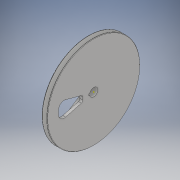
# Autodesk Inventor part: Součást6
Saved by Autodesk Inventor 2019 (Build 230136000, 136)
## iProperties
Created: 2019-10-22
Part Number: Součást6
Material: Všeobecné
Document SubType Name: Modeling
Designer: micaf
Density: 1 g/cm^3
Appearance: Výchozí
Author: micaf
Autodesk Inventor part; units mm, degrees
ref_plane "YZ Plane" through (0, 0, 0) normal (1, 0, 0) x (0, 1, 0)
ref_plane "XY Plane" through (0, 0, 0) normal (0, 0, 1) x (1, 0, 0)
sketch "Náčrt1" plane through (0, 0, 0) normal (0, 0, 1) x (1, 0, 0)
  line L0 (0, -53.3418) -> (0, 320.0509) projected
  line L1 (-48, 0) -> (8, 0) projected
  line L2 (0, 250) -> (0, 0)
  line L3 (0, 0) -> (-40, 0)
  line L4 (-40, 0) -> (-40, 30)
  line L5 (-40, 30) -> (-15, 30)
  line L6 (-15, 30) -> (-15, 210)
  line L7 (-15, 210) -> (-30, 210)
  line L8 (-30, 210) -> (-30, 250)
  line L9 (-26.5993, 250) -> (-17.5, 225)
  line L10 (-17.5, 225) -> (-12.5, 225)
  line L11 (-15, 225) -> (-15, 266.7091) construction
  line L12 (-12.5, 225) -> (-3.4007, 250)
  line L13 (-30, 250) -> (-26.5993, 250)
  line L14 (-3.4007, 250) -> (0, 250)
  dimension "d0" = 30
  dimension "d1" = 40
  dimension "d2" = 15
  dimension "d3" = 250
  dimension "d14" = 30
  dimension "d15" = 15
  dimension "d16" = 20
  dimension "d17" = 20
  dimension "d18" = 25
  dimension "d19" = 40
  dimension "d23" = 5
  dimension "d24" = 15
  constraints: 26 end point, 3 perpendicular, 3 vertical, 2 collinear, 2 horizontal, 2 point on line, 1 midpoint
  measures "d0" distance of L3.end L4.end
  measures "d1" distance of L2.end L3.end
  measures "d2" distance between parallel lines of L2 L6
  measures "d3" distance of L2.start L2.end
  measures "d14" distance of L2.start L8.end
  measures "d15" distance from line of L11 L2.start
  measures "d16" angle of L11 L12
  measures "d17" angle of L9 L11
  measures "d18" vertical distance of L8.end L9.end
  measures "d19" distance of L7.end L8.end
  measures "d23" distance of L9.end L10.end
  measures "d24" distance of L6.end L7.end
revolve "Rotace1" add sketch "Náčrt1" angle 360 about axis through (-10, 0, 0) along (1, 0, 0)
draft "PlochaZešikmení1" angle 10 pull direction (-1, 0, 0) faces at (-31.6667, 29.9027, -2.414) fixed edges at (-40, -30, 0)
draft "PlochaZešikmení2" angle 10 pull direction (1, 0, 0) faces at (-20, 96.0909, -186.7259) fixed edges at (-15, -210, 0)
fillet "Zaoblení1" radius 2 4 edges at (-40, -30, 0) (-17.5, -225, 0) (0, -250, 0) (-30, -250, 0)
fillet "Zaoblení1" radius 5 2 edges at (-15, -34.4082, 0) (-15, -210, 0)
sketch "Náčrt2" plane through (-40, 0, 0) normal (-1, 0, 0) x (0, 0, 1)
  line L0 (0, -350) -> (0, 350) projected
  line L1 (-350, 0) -> (350, 0) projected
  arc A0 (21.4243, 5) -> (21.4243, -5) centre (0, 0) ccw
  line L2 (26, 0) -> (26, 5)
  line L3 (26, 5) -> (21.4243, 5)
  line L4 (26, 0) -> (26, -5)
  line L5 (26, -5) -> (21.4243, -5)
  dimension "d32" = 26
  dimension "d33" = 10
  dimension "d35" = 22
  constraints: 8 end point, 2 point on circle, 2 symmetric about line, 1 centre point, 1 coincident, 1 perpendicular, 1 point on line, 1 vertical
  measures "d32" horizontal distance of L2.end point (0, 0)
  measures "d33" distance of L4.end L2.end
  measures "d35" radius of A0
extrude "Vysunutí1" cut sketch "Náčrt2" against normal through all
sketch "Náčrt3" plane through (0, 0, 0) normal (0, 1, 0) x (-1, 0, 0)
  point P0 (0, 0)
sketch "Náčrt5" plane through (0, 0, 0) normal (1, 0, 0) x (0, 1, 0)
  circle A0 centre (0, 0) radius 204.0412 projected
  circle A1 centre (0, 0) radius 38.6037 projected
  circle A2 centre (0, 0) radius 38.6037 projected
  circle A3 centre (0, 0) radius 204.0412 projected
  circle A4 centre (0, 0) radius 38.6037 projected
  circle A5 centre (0, 0) radius 204.0412 projected
  circle A6 centre (0, 0) radius 207.3551 projected
  arc A7 (15.5291, 57.9555) -> (-15.5291, 57.9555) centre (0, 0) ccw
  arc A8 (49.1756, 183.5259) -> (-49.1756, 183.5259) centre (0, 0) ccw
  circle A9 centre (0, 0) radius 38.6037 projected
  circle A10 centre (0, 0) radius 204.0412 projected
  line L0 (0, 0) -> (0, 190) construction
  line L1 (-350, 0) -> (350, 0) construction
  line L2 (0, -350) -> (0, 350) construction
  line L3 (0, 0) -> (49.1756, 183.5259)
  line L4 (0, 0) -> (-49.1756, 183.5259)
  dimension "d41" = 190
  dimension "d43" = 190
  dimension "d45" = 15
  dimension "d46" = 15
  dimension "d47" = 380
  dimension "d49" = 120
  constraints: 6 end point, 4 point on circle, 2 centre point, 2 coincident, 2 point on line, 1 symmetric about line
  measures "d41" distance of L0.start L0.end
  measures "d43" radius of A8
  measures "d45" angle of L3 L2
  measures "d46" angle of L0 L4
  measures "d47" diameter of A8
  measures "d49" diameter of A7
fillet "Zaoblení2" radius 0.5 2 edges at (-20, 5, 26) (-20, -5, 26)
extrude "Vysunutí2" cut sketch "Náčrt5" against normal through all contours A7 L4 A8 L3
fillet "Zaoblení3" radius 30 2 edges at (-7.5, 49.1756, 183.5259) (-7.5, -49.1756, 183.5259)
fillet "Zaoblení4" radius 10 2 edges at (-7.5, 15.5291, 57.9555) (-7.5, -15.5291, 57.9555)
ref_plane "Pracovní rovina1" through (0, 0, 0) normal (0, 0.8660254, 0.5) x (1, 0, 0)
sketch "Náčrt6" plane through (0, 0, 0) normal (0, 0.8660254, 0.5) x (1, 0, 0)
  line L0 (-38.3473, -30.2914) -> (-19.1318, -33.6796) projected
  line L1 (-20.8682, -208.9653) -> (-30, -207.3551) projected
  line L2 (-30, -207.3551) -> (-30, 207.3551) projected
  line L3 (-38.3473, -30.2914) -> (-30, -207.3551)
  line L4 (-15, -204.0412) -> (-15, 204.0412) projected
  line L5 (-30, -207.3551) -> (-15, -204.0412)
  line L6 (-15, -34.4082) -> (-38.3473, -30.2914)
  line L7 (-15, -34.4082) -> (-15, -204.0412)
  point P0 (0, 0)
  constraints: 8 end point, 1 point on line, 1 vertical
extrude "Vysunutí3" add sketch "Náčrt6" along normal mid plane 10
